# Autodesk Inventor part: DMC2700UDM
Saved by Autodesk Inventor 2016 SP1 (Build 200210100, 210)
## iProperties
Created: 2015-11-19
Part Number: DMC2700UDM
Material: Generic
Document SubType Name: Modeling
Designer: PhillipD
Density: 1 g/cm^3
Appearance: SOT26, DMC2700UDM
Author: PhillipD
Autodesk Inventor part; units mm, degrees
ref_plane "YZ Plane" through (0, 0, 0) normal (1, 0, 0) x (0, 1, 0)
ref_plane "XZ Plane" through (0, 0, 0) normal (0, 1, 0) x (-1, 0, 0)
ref_plane "XY Plane" through (0, 0, 0) normal (0, 0, 1) x (1, 0, 0)
sketch "SOT26, DMC2700UDM_73" plane through (0, 0, 0) normal (0, 0, 1) x (1, 0, 0)
  line L0 (-1.943, 0.8635) -> (1.5635, 0.8635)
  line L1 (1.5635, 0.8635) -> (1.5635, -1.443)
  line L2 (1.5635, -1.443) -> (-1.943, -1.443)
  line L3 (-1.943, -1.443) -> (-1.943, 0.8635)
  constraints: 8 end point
extrude "Extrusion1" add sketch "SOT26, DMC2700UDM_73" along normal blind 1
body "Solid1"
